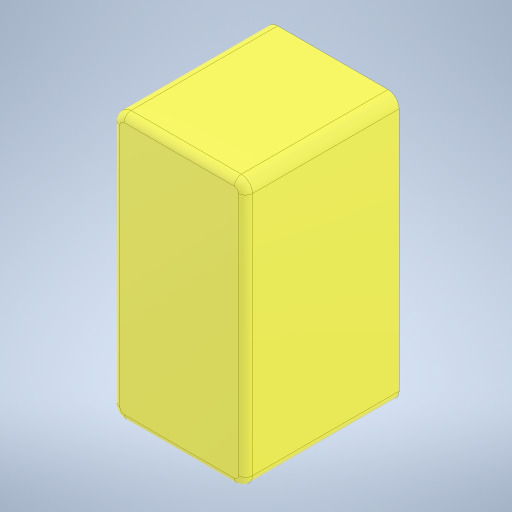
# Autodesk Inventor part: květináč
Saved by Autodesk Inventor 2024 (Build 280153000, 153)
## iProperties
Created: 2025-04-20
Part Number: květináč
Material: Všeobecné
Document SubType Name: Modeling
Designer: annav
Density: 1 g/cm^3
Appearance: Hladká – žlutá
Author: annav
Autodesk Inventor part; units mm, degrees
ref_plane "YZ Plane" through (0, 0, 0) normal (1, 0, 0) x (0, 1, 0)
ref_plane "XZ Plane" through (0, 0, 0) normal (0, 1, 0) x (-1, 0, 0)
ref_plane "XY Plane" through (0, 0, 0) normal (0, 0, 1) x (1, 0, 0)
sketch "Náčrt1" plane through (0, 0, 0) normal (0, 1, 0) x (-1, 0, 0)
  line L0 (0, -133.7) -> (0, 133.7) projected
  line L1 (-66.5, 0) -> (66.5, 0) projected
  line L2 (-47.5, 95.5) -> (47.5, 95.5)
  line L3 (47.5, 95.5) -> (47.5, -95.5)
  line L4 (47.5, -95.5) -> (-47.5, -95.5)
  line L5 (-47.5, -95.5) -> (-47.5, 95.5)
  line L6 (-47.5, 95.5) -> (47.5, -95.5) construction
  line L7 (47.5, 95.5) -> (-47.5, -95.5) construction
  point P0 (0, 0)
  dimension "d0" = 191
  dimension "d1" = 95
  constraints: 12 end point, 2 midpoint, 2 parallel, 1 horizontal, 1 perpendicular
  measures "d0" distance of L2.end L3.end
  measures "d1" distance of L3.end L4.end
extrude "Vysunutí1" add sketch "Náčrt1" along normal blind 110
sketch "Náčrt2" plane through (0, 110, 0) normal (0, 1, 0) x (1, 0, 0)
  line L0 (0, 133.7) -> (0, -133.7) projected
  line L1 (66.5, 0) -> (-66.5, 0) projected
  circle A0 centre (0, -48) radius 42.5
  line L2 (-47.5, -95.5) -> (47.5, -95.5) projected
  point P0 (0, 0)
  dimension "d4" = 85
  dimension "d5" = 47.5
  constraints: 1 centre point, 1 point on line
  measures "d4" diameter of A0
  measures "d5" distance from line of L2 A0.centre
extrude "Vysunutí2" cut sketch "Náčrt2" against normal blind 85
sketch "Náčrt3" plane through (0, 110, 0) normal (0, 1, 0) x (1, 0, 0)
  line L0 (66.5, 0) -> (-66.5, 0) projected
  line L1 (0, 133.7) -> (0, -133.7) projected
  circle A0 centre (0, -48) radius 42.5 projected
  line L2 (-42.5, -0.5) -> (42.5, -0.5)
  line L3 (42.5, -0.5) -> (42.5, 29.5)
  line L4 (42.5, 29.5) -> (-42.5, 29.5)
  line L5 (-42.5, 29.5) -> (-42.5, -0.5)
  point P0 (0, 0)
  dimension "d8" = 30
  dimension "d9" = 85
  dimension "d10" = 47.5
  constraints: 8 end point, 2 parallel, 1 horizontal, 1 perpendicular, 1 other
  measures "d8" distance of L4.end L2.start
  measures "d9" distance of L3.end L4.end
  measures "d10" distance from line of L2 A0.centre
extrude "Vysunutí3" cut sketch "Náčrt3" against normal blind 105 contours L3 L2 L1 L0 | L0 L1 L4 L3 | L1 L2 L5 L0 | L0 L5 L4 L1
sketch "Náčrt4" plane through (0, 110, 0) normal (0, 1, 0) x (1, 0, 0)
  line L0 (0, 133.7) -> (0, -133.7) projected
  line L1 (66.5, 0) -> (-66.5, 0) projected
  line L2 (-42.5, 34.5) -> (42.5, 34.5)
  line L3 (42.5, 34.5) -> (42.5, 84.5)
  line L4 (42.5, 84.5) -> (-42.5, 84.5)
  line L5 (-42.5, 84.5) -> (-42.5, 34.5)
  line L6 (-42.5, 29.5) -> (42.5, 29.5) projected
  point P0 (0, 0)
  dimension "d13" = 5
  dimension "d14" = 50
  dimension "d15" = 85
  constraints: 8 end point, 2 parallel, 1 horizontal, 1 perpendicular, 1 other
  measures "d13" distance between parallel lines of L2 L6
  measures "d14" distance of L4.end L2.start
  measures "d15" distance of L3.end L4.end
extrude "Vysunutí4" cut sketch "Náčrt4" against normal blind 105
sketch "Náčrt6" plane through (0, 25, 48) normal (0, 1, 0) x (1, 0, 0)
  circle A0 centre (0, 0) radius 42.5 projected
  line L0 (66.5, 48) -> (-66.5, 48) projected
  line L1 (0, 181.7) -> (0, -85.7) projected
  circle A1 centre (0, 0) radius 32.5
  point P0 (0, 48)
  dimension "d24" = 65
  constraints: 1 centre point, 1 coincident
  measures "d24" diameter of A1
extrude "Vysunutí6" cut sketch "Náčrt6" against normal blind 10 contours A1 L1 | L1 A1
fillet "Zaoblení1" radius 8 4 edges at (47.5, 55, -95.5) (-47.5, 55, -95.5) (47.5, 55, 95.5) (-47.5, 55, 95.5)
fillet "Zaoblení2" radius 5 8 edges at (45.1569, 0, -93.1569) (0, 0, -95.5) (-45.1569, 0, -93.1569) (-47.5, 0, 0) (-45.1569, 0, 93.1569) (0, 0, 95.5) (45.1569, 0, 93.1569) (47.5, 0, 0)
sketch "Náčrt7" plane through (0, 110, 0) normal (0, 1, 0) x (1, 0, 0)
  line L0 (0, 133.7) -> (0, -133.7) projected
  line L1 (66.5, 0) -> (-66.5, 0) projected
  circle A0 centre (0, -48) radius 42.5 projected
  line L2 (-45.5, -3.5) -> (45.5, -3.5)
  line L3 (45.5, -3.5) -> (45.5, 87.5)
  line L4 (45.5, 87.5) -> (-45.5, 87.5)
  line L5 (-45.5, 87.5) -> (-45.5, -3.5)
  point P0 (0, 0)
  dimension "d29" = 91
  dimension "d30" = 44.5
  dimension "d31" = 91
  constraints: 8 end point, 2 parallel, 1 horizontal, 1 perpendicular, 1 other
  measures "d29" distance between parallel lines of L4 L2
  measures "d30" distance from line of L2 A0.centre
  measures "d31" distance between parallel lines of L3 L5
extrude "Vysunutí7" cut sketch "Náčrt7" against normal blind 3 contours L4 L3 L1 L0 | L0 L1 L5 L4 | L1 L3 L2 L0 | L0 L2 L5 L1
sketch "Náčrt8" plane through (42.5, 5, -34.5) normal (0, 0, -1) x (-1, 0, 0)
  line L0 (85, 102) -> (0, 102) projected
  line L1 (85, 102) -> (85, 0) projected
  circle A0 centre (73, 95) radius 3.5
  point P0 (42.5, -5)
  dimension "d34" = 7
  dimension "d35" = 12
  dimension "d36" = 3.5
  constraints: 1 centre point
  measures "d34" diameter of A0
  measures "d35" distance from line of L1 A0.centre
  measures "d36" distance edge to line of A0 L0
extrude "Vysunutí8" cut sketch "Náčrt8" against normal blind 70
sketch "Náčrt9" plane through (42.5, 5, -34.5) normal (0, 0, -1) x (-1, 0, 0)
  line L0 (85, 102) -> (0, 102) projected
  line L1 (0, 102) -> (0, 0) projected
  line L2 (85, 102) -> (85, 0) projected
  point P0 (42.5, -5)
  point P1 (42.5, 92)
  dimension "d39" = 42.5
  dimension "d40" = 10
  measures "d39" distance from line of L2 point (42.5, 92)
  measures "d40" distance from line of L0 point (42.5, 92)
hole "Díra1" at (0, 97, -34.5) direction (0, 0, 1) diameter 3 depth 8 tip angle 118
sketch "Náčrt10" plane through (42.5, 5, 0.5) normal (0, 0, -1) x (-1, 0, 0)
  line L0 (85, 102) -> (0, 102) projected
  line L1 (0, 102) -> (0, 0) projected
  line L2 (85, 102) -> (85, 0) projected
  circle A0 centre (42.5, 92) radius 1.5 projected
  point P0 (42.5, -5)
  constraints: 1 coincident
hole "Díra2" at (0, 97, 0.5) direction (0, 0, 1) diameter 3 depth 8 tip angle 118
